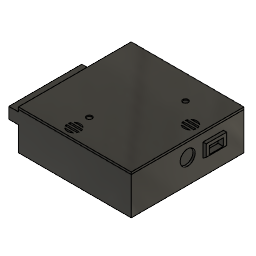
Gabinete Protetor da PCB (Autodesk Fusion 360 design; units mm, degrees)
Autodesk Fusion 360 part; units mm, degrees
(part 1 of 4)
sketch "Esboço1" plane through (0, 0, 1.51) normal (0, 0, 1) x (-1, 0, 0)
  line L0 (-169, 140.5) -> (-269, 140.5)
  line L1 (-269, 140.5) -> (-269, 40.5)
  line L2 (-269, 40.5) -> (-169, 40.5)
  line L3 (-169, 40.5) -> (-169, 140.5)
  circle A0 centre (-173, 132) radius 0.475
  circle A1 centre (-173, 129.5) radius 0.475
  circle A2 centre (-173, 127) radius 0.475
  circle A3 centre (-183, 128.5) radius 0.5
  circle A4 centre (-186.5, 135.5) radius 0.475
  circle A5 centre (-189, 135.5) radius 0.475
  circle A6 centre (-191.5, 135.5) radius 0.475
  circle A7 centre (-194, 135.5) radius 0.475
  circle A8 centre (-185.54, 128.5) radius 0.5
  circle A9 centre (-188.08, 128.5) radius 0.5
  circle A10 centre (-190.62, 128.5) radius 0.5
  circle A11 centre (-193.16, 128.5) radius 0.5
  circle A12 centre (-195.7, 128.5) radius 0.5
  circle A13 centre (-173, 124.5) radius 0.475
  circle A14 centre (-174.608, 114.85) radius 0.5
  circle A15 centre (-183, 119) radius 0.5
  circle A16 centre (-185.54, 119) radius 0.5
  circle A17 centre (-188.08, 119) radius 0.5
  circle A18 centre (-190.62, 119) radius 0.5
  circle A19 centre (-193.16, 119) radius 0.5
  circle A20 centre (-195.7, 119) radius 0.5
  circle A21 centre (-208.9267, 137.648) radius 0.5
  circle A22 centre (-208.9267, 130.048) radius 0.5
  circle A23 centre (-205.994, 118.364) radius 0.45
  circle A24 centre (-207.264, 118.364) radius 0.45
  circle A25 centre (-208.534, 118.364) radius 0.45
  circle A26 centre (-209.804, 118.364) radius 0.45
  circle A27 centre (-174.608, 112.31) radius 0.5
  circle A28 centre (-174.608, 109.77) radius 0.5
  circle A29 centre (-174.608, 107.23) radius 0.5
  circle A30 centre (-174.608, 104.69) radius 0.5
  circle A31 centre (-174.608, 102.15) radius 0.5
  circle A32 centre (-174.608, 99.61) radius 0.5
  circle A33 centre (-174.608, 97.07) radius 0.5
  circle A34 centre (-199.644, 109.474) radius 0.4
  circle A35 centre (-204.724, 109.474) radius 0.4
  circle A36 centre (-209.804, 109.474) radius 0.4
  circle A37 centre (-199.644, 101.854) radius 0.4
  circle A38 centre (-204.724, 101.854) radius 0.4
  circle A39 centre (-209.804, 101.854) radius 0.4
  circle A40 centre (-222, 136.5) radius 1.6
  circle A41 centre (-231.3, 130.015) radius 0.51
  circle A42 centre (-231.3, 127.475) radius 0.51
  circle A43 centre (-223.774, 123.324) radius 0.475
  circle A44 centre (-223.774, 120.824) radius 0.475
  circle A45 centre (-225.774, 124.924) radius 0.6
  circle A46 centre (-223.774, 118.324) radius 0.475
  circle A47 centre (-223.774, 115.824) radius 0.475
  circle A48 centre (-231.3, 124.935) radius 0.51
  circle A49 centre (-231.3, 122.395) radius 0.51
  circle A50 centre (-231.3, 119.855) radius 0.51
  circle A51 centre (-231.3, 117.315) radius 0.51
  circle A52 centre (-231.3, 114.775) radius 0.51
  circle A53 centre (-264.5, 136.5) radius 1.6
  circle A54 centre (-256.7, 130.015) radius 0.51
  circle A55 centre (-256.7, 127.475) radius 0.51
  circle A56 centre (-256.7, 124.935) radius 0.51
  circle A57 centre (-256.7, 122.395) radius 0.51
  circle A58 centre (-263.652, 123.414) radius 0.475
  circle A59 centre (-263.652, 120.914) radius 0.475
  circle A60 centre (-256.7, 119.855) radius 0.51
  circle A61 centre (-256.7, 117.315) radius 0.51
  circle A62 centre (-256.7, 114.775) radius 0.51
  circle A63 centre (-263.652, 118.414) radius 0.475
  circle A64 centre (-263.652, 115.914) radius 0.475
  circle A65 centre (-223.774, 113.324) radius 0.475
  circle A66 centre (-223.774, 110.824) radius 0.475
  circle A67 centre (-223.774, 108.324) radius 0.475
  circle A68 centre (-223.774, 105.824) radius 0.475
  circle A69 centre (-223.774, 103.324) radius 0.475
  circle A70 centre (-231.3, 112.235) radius 0.51
  circle A71 centre (-231.3, 109.695) radius 0.51
  circle A72 centre (-231.3, 107.155) radius 0.51
  circle A73 centre (-231.3, 104.615) radius 0.51
  circle A74 centre (-223.774, 100.824) radius 0.475
  circle A75 centre (-231.3, 102.075) radius 0.51
  circle A76 centre (-231.3, 99.535) radius 0.51
  circle A77 centre (-231.3, 96.995) radius 0.51
  circle A78 centre (-231.3, 94.455) radius 0.51
  circle A79 centre (-256.7, 112.235) radius 0.51
  circle A80 centre (-256.7, 109.695) radius 0.51
  circle A81 centre (-263.652, 113.414) radius 0.475
  circle A82 centre (-263.652, 110.914) radius 0.475
  circle A83 centre (-263.652, 108.414) radius 0.475
  circle A84 centre (-256.7, 107.155) radius 0.51
  circle A85 centre (-256.7, 104.615) radius 0.51
  circle A86 centre (-263.652, 105.914) radius 0.475
  circle A87 centre (-263.652, 103.414) radius 0.475
  circle A88 centre (-256.7, 102.075) radius 0.51
  circle A89 centre (-256.7, 99.535) radius 0.51
  circle A90 centre (-256.7, 96.995) radius 0.51
  circle A91 centre (-263.652, 100.914) radius 0.475
  circle A92 centre (-261.652, 99.314) radius 0.6
  circle A93 centre (-256.7, 94.455) radius 0.51
  circle A94 centre (-182.3, 86.545) radius 0.51
  circle A95 centre (-175.26, 79.68) radius 0.475
  circle A96 centre (-177.26, 81.28) radius 0.6
  circle A97 centre (-182.3, 84.005) radius 0.51
  circle A98 centre (-182.3, 81.465) radius 0.51
  circle A99 centre (-182.3, 78.925) radius 0.51
  circle A100 centre (-175.26, 77.18) radius 0.475
  circle A101 centre (-175.26, 74.68) radius 0.475
  circle A102 centre (-182.3, 76.385) radius 0.51
  circle A103 centre (-182.3, 73.845) radius 0.51
  circle A104 centre (-175.26, 72.18) radius 0.475
  circle A105 centre (-175.26, 69.68) radius 0.475
  circle A106 centre (-175.26, 67.18) radius 0.475
  circle A107 centre (-182.3, 71.305) radius 0.51
  circle A108 centre (-182.3, 68.765) radius 0.51
  circle A109 centre (-207.7, 86.545) radius 0.51
  circle A110 centre (-207.7, 84.005) radius 0.51
  circle A111 centre (-207.7, 81.465) radius 0.51
  circle A112 centre (-207.7, 78.925) radius 0.51
  circle A113 centre (-207.7, 76.385) radius 0.51
  circle A114 centre (-207.7, 73.845) radius 0.51
  circle A115 centre (-214.647, 76.979) radius 0.5
  circle A116 centre (-214.647, 74.439) radius 0.5
  circle A117 centre (-207.7, 71.305) radius 0.51
  circle A118 centre (-207.7, 68.765) radius 0.51
  circle A119 centre (-214.647, 71.899) radius 0.5
  circle A120 centre (-214.647, 69.359) radius 0.5
  circle A121 centre (-214.647, 66.819) radius 0.5
  circle A122 centre (-175.26, 64.68) radius 0.475
  circle A123 centre (-175.26, 62.18) radius 0.475
  circle A124 centre (-182.3, 66.225) radius 0.51
  circle A125 centre (-182.3, 63.685) radius 0.51
  circle A126 centre (-182.3, 61.145) radius 0.51
  circle A127 centre (-175.26, 59.68) radius 0.475
  circle A128 centre (-175.26, 57.18) radius 0.475
  circle A129 centre (-182.3, 58.605) radius 0.51
  circle A130 centre (-182.3, 56.065) radius 0.51
  circle A131 centre (-182.3, 53.525) radius 0.51
  circle A132 centre (-182.3, 50.985) radius 0.51
  circle A133 centre (-174, 44.5) radius 1.6
  circle A134 centre (-207.7, 66.225) radius 0.51
  circle A135 centre (-207.7, 63.685) radius 0.51
  circle A136 centre (-207.7, 61.145) radius 0.51
  circle A137 centre (-214.647, 64.279) radius 0.5
  circle A138 centre (-214.647, 61.739) radius 0.5
  circle A139 centre (-207.7, 58.605) radius 0.51
  circle A140 centre (-207.7, 56.065) radius 0.51
  circle A141 centre (-214.647, 59.199) radius 0.5
  circle A142 centre (-214.647, 56.659) radius 0.5
  circle A143 centre (-207.7, 53.525) radius 0.51
  circle A144 centre (-207.7, 50.985) radius 0.51
  circle A145 centre (-233.68, 76.454) radius 0.4
  circle A146 centre (-238.76, 76.454) radius 0.4
  circle A147 centre (-233.68, 68.834) radius 0.4
  circle A148 centre (-238.76, 68.834) radius 0.4
  circle A149 centre (-243.84, 76.454) radius 0.4
  circle A150 centre (-243.84, 68.834) radius 0.4
  circle A151 centre (-257.058, 77.216) radius 0.5
  circle A152 centre (-264.658, 77.216) radius 0.5
  circle A153 centre (-237.617, 60.452) radius 0.45
  circle A154 centre (-238.887, 60.452) radius 0.45
  circle A155 centre (-240.157, 60.452) radius 0.45
  circle A156 centre (-241.427, 60.452) radius 0.45
  circle A157 centre (-222, 44.5) radius 1.6
  circle A158 centre (-232.022, 43.942) radius 0.475
  circle A159 centre (-234.522, 43.942) radius 0.475
  circle A160 centre (-237.022, 43.942) radius 0.475
  circle A161 centre (-239.522, 43.942) radius 0.475
  circle A162 centre (-257.556, 61.976) radius 0.75
  circle A163 centre (-259.656, 61.976) radius 0.4
  circle A164 centre (-261.656, 61.976) radius 0.4
  circle A165 centre (-263.656, 61.976) radius 0.4
  circle A166 centre (-265.756, 61.976) radius 0.75
  circle A167 centre (-258.318, 54.864) radius 0.7
  circle A168 centre (-263.398, 54.864) radius 0.7
  circle A169 centre (-245.722, 48.224) radius 0.55
  circle A170 centre (-245.722, 43.724) radius 0.55
  circle A171 centre (-252.222, 48.224) radius 0.55
  circle A172 centre (-252.222, 43.724) radius 0.55
  circle A173 centre (-258.826, 47.1575) radius 0.65
  circle A174 centre (-263.826, 47.1575) radius 0.65
  line L4 (-168.5, 141) -> (-269.5, 141)
  line L5 (-269.5, 141) -> (-269.5, 40)
  line L6 (-269.5, 40) -> (-168.5, 40)
  line L7 (-168.5, 40) -> (-168.5, 141)
  line L8 (-166.5, 143) -> (-271.5, 143)
  line L9 (-271.5, 143) -> (-271.5, 38)
  line L10 (-271.5, 38) -> (-166.5, 38)
  line L11 (-166.5, 38) -> (-166.5, 143)
  dimension "d1" = 0.5
  dimension "d2" = 2.5
extrude "Extrusão1" add sketch "Esboço1" along normal blind 15 and the other way blind 4 contours L8 L9 L10 L11 makes body 1
extrude "Extrusão2" add 1 faces at (270.8333, -107.3333, -2.49) along direction (0, 0, -1) blind 7 on bodies 1 bodies 1
sketch "Esboço2" plane through (0, 0, -9.49) normal (0, 0, -1) x (1, 0, 0)
  line L0 (168.5, 40) -> (168.5, 141)
  line L1 (168.5, 141) -> (269.5, 141)
  line L2 (269.5, 141) -> (269.5, 40)
  line L3 (269.5, 40) -> (168.5, 40)
  line L4 (166.5, 143) -> (166.5, 38)
  line L5 (166.5, 38) -> (271.5, 38)
  line L6 (271.5, 38) -> (271.5, 143)
  line L7 (271.5, 143) -> (166.5, 143)
extrude "Extrusão3" add sketch "Esboço2" along normal blind 2 contours L0 L1 L2 L3 | L4 L5 L6 L7 bodies 1
sketch "Esboço3" plane through (0, 0, -9.49) normal (0, 0, 1) x (-1, 0, 0)
  line L0 (-168.5, 141) -> (-269.5, 141)
  line L1 (-269.5, 141) -> (-269.5, 40)
  line L2 (-269.5, 40) -> (-168.5, 40)
  line L3 (-168.5, 40) -> (-168.5, 141)
  circle A0 centre (-174, 44.5) radius 1.6
  circle A1 centre (-264.5, 136.5) radius 1.6
  circle A2 centre (-222, 136.5) radius 1.6
  circle A3 centre (-222, 44.5) radius 1.6
extrude "Extrusão4" add sketch "Esboço3" along normal blind 15 contours A0 | A1 | A2 | A3 bodies 1
sketch "Esboço4" plane through (0, 0, -9.49) normal (0, 0, 1) x (-1, 0, 0)
  circle A0 centre (-264.5, 136.5) radius 1.6
  circle A1 centre (-174, 44.5) radius 1.6
  circle A2 centre (-222, 136.5) radius 1.6
  circle A3 centre (-222, 44.5) radius 1.6
  line L0 (-168.5, 141) -> (-269.5, 141)
  line L1 (-269.5, 141) -> (-269.5, 40)
  line L2 (-269.5, 40) -> (-168.5, 40)
  line L3 (-168.5, 40) -> (-168.5, 141)
  circle A4 centre (-174, 44.5) radius 3.6
  circle A5 centre (-222, 44.5) radius 3.6
  circle A6 centre (-222, 136.5) radius 3.6
  circle A7 centre (-264.5, 136.5) radius 3.6
  dimension "d13" = 2
  dimension "d14" = 2
  dimension "d15" = 2
  dimension "d16" = 2
extrude "Extrusão5" add sketch "Esboço4" along normal blind 9.5 contours A4 | A5 | A6 | A7 bodies 1
sketch "Esboço5" plane through (0, -38, 0) normal (0, 1, 0) x (-1, 0, 0)
  line L0 (-166.5, -11.49) -> (-166.5, 16.51)
  line L1 (-166.5, 16.51) -> (-271.5, 16.51)
  line L2 (-271.5, 16.51) -> (-271.5, -11.49)
  line L3 (-271.5, -11.49) -> (-166.5, -11.49)
  line L4 (-266.406, 12.4324) -> (-256.246, 12.4324)
  line L5 (-256.246, 12.4324) -> (-256.246, 2.595)
  line L6 (-256.246, 2.595) -> (-266.406, 2.595)
  line L7 (-266.406, 2.595) -> (-266.406, 12.4324)
  point P0 (-266.406, 12.4324)
  point P1 (-256.246, 12.4324)
  point P2 (-256.246, 2.595)
  point P3 (-266.406, 2.595)
  constraint horizontal L4
  constraint vertical L5
  constraint horizontal L6
  constraint vertical L7
  constraint coincident P2 L5.end
  constraint coincident P0 L4.start
extrude "Extrusão6" cut sketch "Esboço5" against normal blind 7 contours L4 L5 L6 L7 bodies 1
sketch "Esboço6" plane through (0, 0, 16.51) normal (0, 0, 1) x (-1, 0, 0)
  line L0 (-168.5, 141) -> (-168.5, 40)
  line L1 (-168.5, 40) -> (-269.5, 40)
  line L2 (-269.5, 40) -> (-269.5, 141)
  line L3 (-269.5, 141) -> (-168.5, 141)
  line L4 (-166.5, 38) -> (-166.5, 143)
  line L5 (-166.5, 143) -> (-271.5, 143)
  line L6 (-271.5, 143) -> (-271.5, 38)
  line L7 (-271.5, 38) -> (-166.5, 38)
  circle A0 centre (-239.522, 60.452) radius 2.5
  circle A1 centre (-207.899, 118.364) radius 2.5
  circle A2 centre (-208.9267, 133.848) radius 6
  circle A3 centre (-260.858, 77.216) radius 6
  line L8 (-257.756, 60.626) -> (-257.756, 63.326)
  line L9 (-257.756, 63.326) -> (-257.806, 63.326)
  line L10 (-257.806, 63.326) -> (-257.806, 63.726)
  line L11 (-257.806, 63.726) -> (-265.506, 63.726)
  line L12 (-265.506, 63.726) -> (-265.506, 63.326)
  line L13 (-265.506, 63.326) -> (-265.556, 63.326)
  line L14 (-265.556, 63.326) -> (-265.556, 60.626)
  line L15 (-265.556, 60.626) -> (-265.506, 60.626)
  line L16 (-265.506, 60.626) -> (-265.506, 60.226)
  line L17 (-265.506, 60.226) -> (-257.806, 60.226)
  line L18 (-257.806, 60.226) -> (-257.806, 60.626)
  line L19 (-257.806, 60.626) -> (-257.756, 60.626)
  line L20 (-259.656, 62.976) -> (-259.656, 60.976)
  line L21 (-259.656, 60.976) -> (-263.656, 60.976)
  line L22 (-263.656, 60.976) -> (-263.656, 62.976)
  line L23 (-263.656, 62.976) -> (-259.656, 62.976)
extrude "Extrusão7" add sketch "Esboço6" along normal blind 2 separate body contours L0 L1 L2 L3 | L4 L5 L6 L7 makes body 2
sketch "Esboço7" plane through (0, 0, 18.51) normal (0, 0, 1) x (-1, 0, 0)
  circle A0 centre (-260.858, 77.216) radius 6
  circle A1 centre (-207.899, 118.364) radius 2.5
  circle A2 centre (-239.522, 60.452) radius 2.5
  circle A3 centre (-208.9267, 133.848) radius 6
  line L0 (-257.756, 60.626) -> (-257.806, 60.626)
  line L1 (-257.806, 60.626) -> (-257.806, 60.226)
  line L2 (-257.806, 60.226) -> (-265.506, 60.226)
  line L3 (-265.506, 60.226) -> (-265.506, 60.626)
  line L4 (-265.506, 60.626) -> (-265.556, 60.626)
  line L5 (-265.556, 60.626) -> (-265.556, 63.326)
  line L6 (-265.556, 63.326) -> (-265.506, 63.326)
  line L7 (-265.506, 63.326) -> (-265.506, 63.726)
  line L8 (-265.506, 63.726) -> (-257.806, 63.726)
  line L9 (-257.806, 63.726) -> (-257.806, 63.326)
  line L10 (-257.806, 63.326) -> (-257.756, 63.326)
  line L11 (-257.756, 63.326) -> (-257.756, 60.626)
  line L12 (-271.5, 38) -> (-166.5, 38)
  line L13 (-166.5, 38) -> (-166.5, 143)
  line L14 (-166.5, 143) -> (-271.5, 143)
  line L15 (-271.5, 143) -> (-271.5, 38)
  line L16 (-266.858, 77.216) -> (-254.858, 77.216)
  line L17 (-266.858, 76.216) -> (-254.858, 76.216)
  line L18 (-266.858, 78.216) -> (-254.858, 78.216)
  line L19 (-266.858, 79.716) -> (-254.858, 79.716)
  line L20 (-266.858, 81.716) -> (-254.858, 81.716)
  line L21 (-266.858, 72.716) -> (-254.858, 72.716)
  line L22 (-266.858, 74.716) -> (-254.858, 74.716)
  line L23 (-266.858, 69.216) -> (-254.858, 69.216)
  line L24 (-266.858, 71.216) -> (-254.858, 71.216)
  line L25 (-214.9267, 138.348) -> (-202.9267, 138.348)
  line L26 (-214.9267, 136.348) -> (-202.9267, 136.348)
  line L27 (-214.9267, 134.848) -> (-202.9267, 134.848)
  line L28 (-214.9267, 132.848) -> (-202.9267, 132.848)
  line L29 (-214.9267, 131.348) -> (-202.9267, 131.348)
  line L30 (-214.9267, 129.348) -> (-202.9267, 129.348)
  dimension "d23" = 1
  dimension "d24" = -1
  dimension "d27" = 0
  dimension "d28" = -7
  constraint coincident A0 L16.start
  constraint coincident A0 L16.end
  constraint horizontal L16
extrude "Extrusão8" add sketch "Esboço7" against normal blind 2 contours A0 L16 L18 | A0 L16 L17 | A0 L19 L20 | A0 L21 L22 | A3 L27 L28 | A3 L25 L26 | A3 L29 L30 bodies 2
sketch "Esboço8" plane through (0, 0, 16.51) normal (0, 0, -1) x (1, 0, 0)
  arc A0 (254.9419, 76.216) -> (255.4036, 74.716) centre (260.858, 77.216) ccw
  line L0 (254.9419, 76.216) -> (266.7741, 76.216)
  arc A1 (266.3124, 74.716) -> (266.7741, 76.216) centre (260.858, 77.216) ccw
  line L1 (266.3124, 74.716) -> (255.4036, 74.716)
  arc A2 (203.4723, 136.348) -> (203.0106, 134.848) centre (208.9267, 133.848) ccw
  line L2 (203.4723, 136.348) -> (214.381, 136.348)
  arc A3 (214.8427, 134.848) -> (214.381, 136.348) centre (208.9267, 133.848) ccw
  line L3 (214.8427, 134.848) -> (203.0106, 134.848)
  line L4 (203.0106, 132.848) -> (214.8427, 132.848)
  arc A4 (214.381, 131.348) -> (214.8427, 132.848) centre (208.9267, 133.848) ccw
  line L5 (214.381, 131.348) -> (203.4723, 131.348)
  arc A5 (203.0106, 132.848) -> (203.4723, 131.348) centre (208.9267, 133.848) ccw
  arc A6 (255.4036, 79.716) -> (254.9419, 78.216) centre (260.858, 77.216) ccw
  line L6 (255.4036, 79.716) -> (266.3124, 79.716)
  arc A7 (266.7741, 78.216) -> (266.3124, 79.716) centre (260.858, 77.216) ccw
  line L7 (266.7741, 78.216) -> (254.9419, 78.216)
  arc A8 (212.8953, 138.348) -> (204.958, 138.348) centre (208.9267, 133.848) ccw
  line L8 (212.8953, 138.348) -> (204.958, 138.348)
  arc A9 (264.8266, 81.716) -> (256.8894, 81.716) centre (260.858, 77.216) ccw
  line L9 (264.8266, 81.716) -> (256.8894, 81.716)
  line L10 (256.8894, 72.716) -> (264.8266, 72.716)
  arc A10 (256.8894, 72.716) -> (264.8266, 72.716) centre (260.858, 77.216) ccw
  circle A11 centre (207.899, 118.364) radius 2.5
  circle A12 centre (239.522, 60.452) radius 2.5
  line L11 (204.958, 129.348) -> (212.8953, 129.348)
  arc A13 (204.958, 129.348) -> (212.8953, 129.348) centre (208.9267, 133.848) ccw
  line L12 (257.806, 60.626) -> (257.756, 60.626)
  line L13 (257.756, 60.626) -> (257.756, 63.326)
  line L14 (257.756, 63.326) -> (257.806, 63.326)
  line L15 (257.806, 63.326) -> (257.806, 63.726)
  line L16 (257.806, 63.726) -> (265.506, 63.726)
  line L17 (265.506, 63.726) -> (265.506, 63.326)
  line L18 (265.506, 63.326) -> (265.556, 63.326)
  line L19 (265.556, 63.326) -> (265.556, 60.626)
  line L20 (265.556, 60.626) -> (265.506, 60.626)
  line L21 (265.506, 60.626) -> (265.506, 60.226)
  line L22 (265.506, 60.226) -> (257.806, 60.226)
  line L23 (257.806, 60.226) -> (257.806, 60.626)
  line L24 (166.5, 38) -> (271.5, 38)
  line L25 (271.5, 38) -> (271.5, 143)
  line L26 (271.5, 143) -> (166.5, 143)
  line L27 (166.5, 143) -> (166.5, 38)
  line L28 (232.022, 52.952) -> (247.022, 52.952)
  line L29 (247.022, 52.952) -> (247.022, 67.952)
  line L30 (247.022, 67.952) -> (232.022, 67.952)
  line L31 (232.022, 67.952) -> (232.022, 52.952)
  line L32 (232.022, 52.952) -> (247.022, 67.952) construction
  line L33 (247.022, 52.952) -> (232.022, 67.952) construction
  line L34 (215.399, 110.864) -> (215.399, 125.864)
  line L35 (215.399, 125.864) -> (200.399, 125.864)
  line L36 (200.399, 125.864) -> (200.399, 110.864)
  line L37 (200.399, 110.864) -> (215.399, 110.864)
  point P0 (239.522, 60.452)
  dimension "d31" = 15
  dimension "d32" = 15
  dimension "d33" = 15
  dimension "d34" = 15
  constraint horizontal L28
  constraint perpendicular L28 L29
  constraint parallel L28 L30
  constraint parallel L29 L31
  constraint coincident L32 P0
  constraint coincident L33 P0
  constraint coincident P0 A12.centre
  constraint horizontal L37
  constraint perpendicular L34 L37
  constraint parallel L35 L37
  constraint parallel L34 L36
  measures "d31" distance of L29.end L30.end
  measures "d32" distance of L28.end L29.end
  measures "d33" distance of L35.end L34.end
  measures "d34" distance of L34.start L34.end
extrude "Extrusão9" cut sketch "Esboço8" against normal blind 1 contours L28 L29 L30 L31 | L34 L35 L36 L37 bodies 2
extrude "Extrusão10" add 1 faces at (270.8333, -107.3333, 16.51) along direction (0, 0, 1) blind 7 on bodies 1 bodies 1
move_body "Mover1" bodies 2 to x (1, 0, 0) y (0, 1, 0) z (0, 0, 1) at (0, 0, 7)
sketch "Esboço9" plane through (0, 0, 23.51) normal (0, 0, -1) x (1, 0, 0)
  line L0 (166.5, 38) -> (271.5, 38)
  line L1 (271.5, 38) -> (271.5, 143)
  line L2 (271.5, 143) -> (166.5, 143)
  line L3 (166.5, 143) -> (166.5, 38)
  line L4 (257.806, 60.626) -> (257.756, 60.626)
  line L5 (257.756, 60.626) -> (257.756, 63.326)
  line L6 (257.756, 63.326) -> (257.806, 63.326)
  line L7 (257.806, 63.326) -> (257.806, 63.726)
  line L8 (257.806, 63.726) -> (265.506, 63.726)
  line L9 (265.506, 63.726) -> (265.506, 63.326)
  line L10 (265.506, 63.326) -> (265.556, 63.326)
  line L11 (265.556, 63.326) -> (265.556, 60.626)
  line L12 (265.556, 60.626) -> (265.506, 60.626)
  line L13 (265.506, 60.626) -> (265.506, 60.226)
  line L14 (265.506, 60.226) -> (257.806, 60.226)
  line L15 (257.806, 60.226) -> (257.806, 60.626)
  line L16 (204.958, 129.348) -> (212.8953, 129.348)
  arc A0 (204.958, 129.348) -> (212.8953, 129.348) centre (208.9267, 133.848) ccw
  line L17 (256.8894, 72.716) -> (264.8266, 72.716)
  arc A1 (256.8894, 72.716) -> (264.8266, 72.716) centre (260.858, 77.216) ccw
  arc A2 (264.8266, 81.716) -> (256.8894, 81.716) centre (260.858, 77.216) ccw
  line L18 (264.8266, 81.716) -> (256.8894, 81.716)
  arc A3 (212.8953, 138.348) -> (204.958, 138.348) centre (208.9267, 133.848) ccw
  line L19 (212.8953, 138.348) -> (204.958, 138.348)
  arc A4 (255.4036, 79.716) -> (254.9419, 78.216) centre (260.858, 77.216) ccw
  line L20 (255.4036, 79.716) -> (266.3124, 79.716)
  arc A5 (266.7741, 78.216) -> (266.3124, 79.716) centre (260.858, 77.216) ccw
  line L21 (266.7741, 78.216) -> (254.9419, 78.216)
  line L22 (203.0106, 132.848) -> (214.8427, 132.848)
  arc A6 (214.381, 131.348) -> (214.8427, 132.848) centre (208.9267, 133.848) ccw
  line L23 (214.381, 131.348) -> (203.4723, 131.348)
  arc A7 (203.0106, 132.848) -> (203.4723, 131.348) centre (208.9267, 133.848) ccw
  arc A8 (203.4723, 136.348) -> (203.0106, 134.848) centre (208.9267, 133.848) ccw
  line L24 (203.4723, 136.348) -> (214.381, 136.348)
  arc A9 (214.8427, 134.848) -> (214.381, 136.348) centre (208.9267, 133.848) ccw
  line L25 (214.8427, 134.848) -> (203.0106, 134.848)
  arc A10 (254.9419, 76.216) -> (255.4036, 74.716) centre (260.858, 77.216) ccw
  line L26 (254.9419, 76.216) -> (266.7741, 76.216)
  arc A11 (266.3124, 74.716) -> (266.7741, 76.216) centre (260.858, 77.216) ccw
  line L27 (266.3124, 74.716) -> (255.4036, 74.716)
  line L28 (215.399, 125.864) -> (215.399, 110.864)
  line L29 (215.399, 110.864) -> (200.399, 110.864)
  line L30 (200.399, 110.864) -> (200.399, 125.864)
  line L31 (200.399, 125.864) -> (215.399, 125.864)
  line L32 (247.022, 52.952) -> (232.022, 52.952)
  line L33 (232.022, 52.952) -> (232.022, 67.952)
  line L34 (232.022, 67.952) -> (247.022, 67.952)
  line L35 (247.022, 67.952) -> (247.022, 52.952)
  line L36 (269, 40.5) -> (269, 140.5)
  line L37 (269, 140.5) -> (169, 140.5)
  line L38 (169, 140.5) -> (169, 40.5)
  line L39 (169, 40.5) -> (269, 40.5)
  line L40 (267.5, 42) -> (267.5, 139)
  line L41 (267.5, 139) -> (170.5, 139)
  line L42 (170.5, 139) -> (170.5, 42)
  line L43 (170.5, 42) -> (267.5, 42)
  dimension "d39" = -2.5
  dimension "d40" = -4
extrude "Extrusão11" add sketch "Esboço9" along normal blind 10 contours L36 L37 L38 L39 bodies 2
sketch "Esboço10" plane through (166.5, 0, 0) normal (-1, 0, 0) x (0, -1, 0)
  line L0 (143, -11.49) -> (143, 23.51)
  line L1 (143, 23.51) -> (38, 23.51)
  line L2 (38, 23.51) -> (38, -11.49)
  line L3 (38, -11.49) -> (143, -11.49)
  circle A0 centre (90.5, 11.01) radius 7
  dimension "d43" = 14
  measures "d43" diameter of A0
extrude "Extrusão12" cut sketch "Esboço10" against normal blind 35 contours A0 bodies 1 2
sketch "Esboço11" plane through (166.5, 0, 0) normal (-1, 0, 0) x (0, -1, 0)
  line L0 (38, 23.51) -> (143, 23.51)
  line L1 (143, 23.51) -> (143, 25.51)
  line L2 (143, 25.51) -> (38, 25.51)
  line L3 (38, 25.51) -> (38, 23.51)
  line L4 (143, 25.51) -> (146.8418, 28.7101)
  circle A0 centre (144.9209, 27.11) radius 2.5
  line L5 (143, 23.51) -> (145.9431, 24.8285)
  line L6 (139.5, 25.5) -> (143.223, 28.945)
  circle A1 centre (144.9209, 27.11) radius 0.65
  dimension "d46" = 5
  dimension "d47" = 1.3
  constraint coincident L1.end L2.start
  constraint midpoint L4 A0.centre
  constraint coincident L1.end A0
  constraint coincident L0.end L1.start
  constraint coincident A0 L5.end
  constraint tangent A0 L5
  constraint coincident A0 L6.end
  constraint tangent A0 L6
  constraint concentric A0 A1
  measures "d46" distance of L1.end L4.end
  measures "d47" diameter of A1
extrude "Extrusão13" add sketch "Esboço11" against normal blind 10 separate body contours L1 A0 L5 | L4 A0 A1 | L2 A0 L6 | L4 A0 A1 makes body 3
sketch "Esboço12" plane through (166.5, 0, 0) normal (-1, 0, 0) x (0, -1, 0)
  circle A0 centre (90.5, 11.01) radius 7
  line L0 (143, -11.49) -> (143, 23.51)
  line L1 (143, 23.51) -> (38, 23.51)
  line L2 (38, 23.51) -> (38, -11.49)
  line L3 (38, -11.49) -> (143, -11.49)
  circle A1 centre (144.9209, 27.11) radius 0.65
  arc A2 (145.9431, 24.8285) -> (143.223, 28.945) centre (144.9209, 27.11) ccw
  line L4 (144.9209, 29.61) -> (143, 29.61)
  line L5 (143, 29.61) -> (143, 23.51)
  line L6 (143, 23.51) -> (143, 18.51)
  line L7 (143, 18.51) -> (147.1059, 25.8952)
  dimension "d50" = 1.3
  dimension "d51" = 5
  constraint concentric A1 A2
  constraint coincident A2 L4.start
  constraint tangent A2 L4
  constraint perpendicular L0 L4
  constraint coincident L0.end L1.start
  constraint perpendicular L1 L5
  constraint perpendicular L1 L6
  constraint coincident A2 L7.end
  constraint tangent A2 L7
  measures "d50" diameter of A1
  measures "d51" distance of L0.end L6.end
extrude "Extrusão14" add sketch "Esboço12" against normal blind 10 separate body contours L0 A2 L4 L5 L6 L7 makes body 4
move_body "Mover2" bodies 4 to x (1, 0, 0) y (0, 1, 0) z (0, 0, 1) at (10.5, 0, 0)
copy_body "Copiar e colar corpos1" bodies 4 3 makes body 5 makes body 6
move_body "Mover3" bodies 5 6 to x (1, 0, 0) y (0, 1, 0) z (0, 0, 1) at (84.5, 0, 0)
sketch "Esboço13" plane through (0, 0, -9.49) normal (0, 0, 1) x (-1, 0, 0)
  circle A0 centre (-264.5, 136.5) radius 3.6
  circle A1 centre (-174, 44.5) radius 3.6
  circle A2 centre (-222, 136.5) radius 3.6
  circle A3 centre (-222, 44.5) radius 3.6
  line L0 (-168.5, 141) -> (-269.5, 141)
  line L1 (-269.5, 141) -> (-269.5, 40)
  line L2 (-269.5, 40) -> (-168.5, 40)
  line L3 (-168.5, 40) -> (-168.5, 141)
sketch "Esboço14" plane through (271.5, 0, 0) normal (1, 0, 0) x (0, 1, 0)
  circle A0 centre (-144.9209, 27.11) radius 0.65
  line L0 (-147.1059, 25.8952) -> (-143, 18.51)
  line L1 (-143, 18.51) -> (-143, 29.61)
  line L2 (-143, 29.61) -> (-144.9209, 29.61)
  arc A1 (-144.9209, 29.61) -> (-147.1059, 25.8952) centre (-144.9209, 27.11) ccw
  circle A2 centre (-144.9209, 27.11) radius 1
  dimension "d54" = 2
  constraint concentric A0 A2
  measures "d54" diameter of A2
extrude "Extrusão15" cut sketch "Esboço14" against normal blind 130 contours A2 bodies 3 4 5 6
sketch "Esboço15" plane through (0, -38, 0) normal (0, 1, 0) x (-1, 0, 0)
  line L0 (-256.246, 12.4324) -> (-256.246, 2.595)
  line L1 (-256.246, 2.595) -> (-266.406, 2.595)
  line L2 (-266.406, 2.595) -> (-266.406, 12.4324)
  line L3 (-266.406, 12.4324) -> (-256.246, 12.4324)
  line L4 (-166.5, -11.49) -> (-166.5, 23.51)
  line L5 (-166.5, 23.51) -> (-271.5, 23.51)
  line L6 (-271.5, 23.51) -> (-271.5, -11.49)
  line L7 (-271.5, -11.49) -> (-166.5, -11.49)
extrude "Extrusão16" add sketch "Esboço15" against normal blind 2 contours L0 L1 L2 L3 bodies 1
sketch "Esboço16" plane through (166.5, 0, 0) normal (-1, 0, 0) x (0, -1, 0)
  circle A0 centre (90.5, 11.01) radius 7
  line L0 (143, -11.49) -> (143, 23.51)
  line L1 (143, 23.51) -> (38, 23.51)
  line L2 (38, 23.51) -> (38, -11.49)
  line L3 (38, -11.49) -> (143, -11.49)
extrude "Extrusão17" cut sketch "Esboço16" against normal blind 180 contours A0 bodies 1
sketch "Esboço17" plane through (166.5, 0, 0) normal (-1, 0, 0) x (0, -1, 0)
  circle A0 centre (90.5, 11.01) radius 7
  line L0 (143, -11.49) -> (143, 23.51)
  line L1 (143, 23.51) -> (38, 23.51)
  line L2 (38, 23.51) -> (38, -11.49)
  line L3 (38, -11.49) -> (143, -11.49)
extrude "Extrusão18" add sketch "Esboço17" against normal blind 2 contours A0 bodies 1
sketch "Esboço18" plane through (168.5, 0, 0) normal (1, 0, 0) x (0, 1, 0)
  line L0 (-40, -9.49) -> (-40, 23.51)
  line L1 (-40, 23.51) -> (-141, 23.51)
  line L2 (-141, 23.51) -> (-141, -9.49)
  line L3 (-141, -9.49) -> (-40, -9.49)
  line L4 (-134.45, 18.595) -> (-122.05, 18.595)
  line L5 (-122.05, 8.595) -> (-134.45, 8.595)
  line L6 (-119.75, 18.595) -> (-136.75, 18.595)
  line L7 (-136.75, 18.595) -> (-136.75, 8.595)
  line L8 (-136.75, 8.595) -> (-119.75, 8.595)
  line L9 (-119.75, 8.595) -> (-119.75, 18.595)
  line L10 (-119.75, 18.595) -> (-136.75, 8.595) construction
  line L11 (-136.75, 18.595) -> (-119.75, 8.595) construction
  line L12 (-134.45, 8.595) -> (-134.45, 9.9479)
  line L13 (-134.45, 17.2421) -> (-134.45, 18.595)
  line L14 (-134.45, 8.595) -> (-134.45, 9.9479)
  line L15 (-134.45, 17.2421) -> (-134.45, 18.595)
  line L16 (-122.05, 18.595) -> (-122.05, 17.2421)
  line L17 (-122.05, 9.9479) -> (-122.05, 8.595)
  point P0 (-134.45, 8.595)
  point P1 (-122.05, 8.595)
  point P2 (-128.25, 13.595)
  dimension "d63" = 10
  dimension "d64" = 17
  constraint coincident P0 L5.end
  constraint vertical L14
  constraint horizontal L4
  constraint vertical L16
  constraint horizontal L5
  constraint vertical L12
  constraint coincident P1 L5.start
  constraint horizontal L6
  constraint perpendicular L6 L7
  constraint parallel L6 L8
  constraint parallel L7 L9
  constraint coincident L10 P2
  constraint coincident L11 P2
  constraint coincident L10 L12.end
  constraint coincident L11 L13.start
  constraint collinear L12 L13
  constraint collinear L14 L15
  constraint coincident L10 L16.end
  constraint coincident L11 L17.start
  constraint collinear L16 L17
  measures "d63" distance of P0 L4.start
  measures "d64" distance of L7.end L8.end
extrude "Extrusão19" cut sketch "Esboço18" against normal blind 19 contours L4 L5 L6 L7 L8 L9 bodies 1
sketch "Esboço19" plane through (166.5, 0, 0) normal (-1, 0, 0) x (0, -1, 0)
  line L0 (119.75, 18.595) -> (136.75, 18.595)
  line L1 (136.75, 18.595) -> (136.75, 8.595)
  line L2 (136.75, 8.595) -> (119.75, 8.595)
  line L3 (119.75, 8.595) -> (119.75, 18.595)
  line L4 (143, -11.49) -> (143, 23.51)
  line L5 (143, 23.51) -> (38, 23.51)
  line L6 (38, 23.51) -> (38, -11.49)
  line L7 (38, -11.49) -> (143, -11.49)
  line L8 (77, 19.5) -> (97, 19.5)
  line L9 (97, 19.5) -> (97, 2.5)
  line L10 (97, 2.5) -> (77, 2.5)
  line L11 (77, 2.5) -> (77, 19.5)
  line L12 (77, 19.5) -> (97, 2.5) construction
  line L13 (97, 19.5) -> (77, 2.5) construction
  line L14 (99, 0.5) -> (75, 0.5)
  line L15 (75, 0.5) -> (75, 21.5)
  line L16 (75, 21.5) -> (99, 21.5)
  line L17 (99, 21.5) -> (99, 0.5)
  point P0 (87, 11)
  dimension "d67" = 20
  dimension "d68" = 17
  dimension "d69" = -2
  constraint horizontal L8
  constraint perpendicular L8 L9
  constraint parallel L8 L10
  constraint parallel L9 L11
  constraint coincident L12 P0
  constraint coincident L13 P0
  measures "d67" distance of L9.end L10.end
  measures "d68" distance of L8.end L9.end
extrude "Extrusão20" add sketch "Esboço19" along normal blind 7 separate body contours L14 L15 L16 L17 makes body 7
sketch "Esboço20" plane through (159.5, 0, 0) normal (-1, 0, 0) x (0, -1, 0)
  line L0 (97, 2.5) -> (77, 2.5)
  line L1 (77, 2.5) -> (77, 19.5)
  line L2 (77, 19.5) -> (97, 19.5)
  line L3 (97, 19.5) -> (97, 2.5)
  line L4 (99, 21.5) -> (75, 21.5)
  line L5 (75, 21.5) -> (75, 0.5)
  line L6 (75, 0.5) -> (99, 0.5)
  line L7 (99, 0.5) -> (99, 21.5)
  line L8 (75, 21.5) -> (99, 21.5)
  line L9 (99, 21.5) -> (99, 0.5)
  line L10 (99, 0.5) -> (75, 0.5)
  line L11 (75, 0.5) -> (75, 21.5)
  line L12 (89, 11) -> (90, 11)
  line L13 (85, 16) -> (85, 6)
  line L14 (89, 16) -> (89, 6)
  arc A0 (89, 16) -> (85, 16) centre (87, 16) ccw
  arc A1 (85, 6) -> (89, 6) centre (87, 6) ccw
  line L15 (83, 16) -> (83, 6)
  arc A2 (83, 16) -> (79, 16) centre (81, 16) ccw
  line L16 (79, 16) -> (79, 6)
  arc A3 (79, 6) -> (83, 6) centre (81, 6) ccw
  line L17 (95, 16) -> (95, 6)
  arc A4 (95, 16) -> (91, 16) centre (93, 16) ccw
  line L18 (91, 16) -> (91, 6)
  arc A5 (91, 6) -> (95, 6) centre (93, 6) ccw
  dimension "d73" = 4
  dimension "d76" = 6
  dimension "d77" = 0
  constraint horizontal L8
  constraint vertical L9
  constraint horizontal L10
  constraint vertical L11
  constraint coincident L6.end L7.start
  constraint coincident L4.end L5.start
  constraint symmetric L12 A0 A1
  constraint tangent L13 A1
  constraint tangent L14 A1
  constraint coincident L14 L12.start
  measures "d73" diameter of A0
extrude "Extrusão21" add sketch "Esboço20" along normal blind 2 contours L0 L1 L2 L3 | L4 L5 L6 L7 L8 L9 L10 L11 bodies 7
extrude "Extrusão22" cut 1 faces at (164.1667, -97, 13.8333) along direction (0, -1, 0) blind 8 on bodies 7 bodies 7